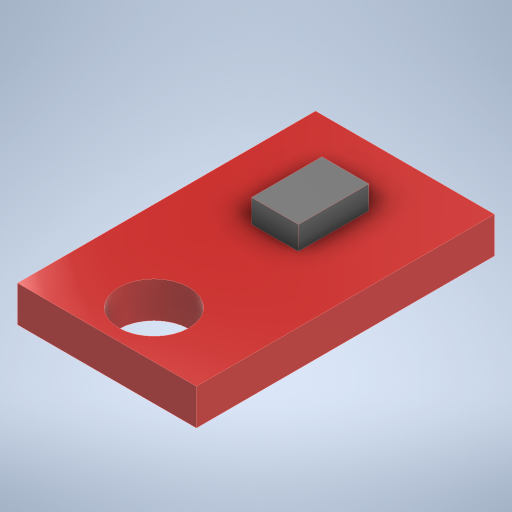
# Autodesk Inventor part: lightSensor
Saved by Autodesk Inventor 2024 (Build 280153000, 153)
## iProperties
Created: 2023-10-20
Part Number: lightSensor
Material: Generic
Document SubType Name: Modeling
Designer: kdcao
Density: 1 g/cm^3
Appearance: Orange-Red
Author: kdcao
Autodesk Inventor part; units mm, degrees
ref_plane "YZ Plane" through (0, 0, 0) normal (1, 0, 0) x (0, 1, 0)
ref_plane "XZ Plane" through (0, 0, 0) normal (0, 1, 0) x (-1, 0, 0)
ref_plane "XY Plane" through (0, 0, 0) normal (0, 0, 1) x (1, 0, 0)
sketch "Sketch1" plane through (0, 0, 0) normal (0, 1, 0) x (-1, 0, 0)
  line L0 (-3.81, 6.35) -> (3.81, 6.35)
  line L1 (3.81, 6.35) -> (3.81, -6.35)
  line L2 (3.81, -6.35) -> (-3.81, -6.35)
  line L3 (-3.81, -6.35) -> (-3.81, 6.35)
  line L4 (-3.81, 6.35) -> (3.81, -6.35) construction
  line L5 (3.81, 6.35) -> (-3.81, -6.35) construction
  point P0 (0, 0)
  dimension "d0" = 12.7
  dimension "d1" = 7.62
  constraints: 12 end point, 2 midpoint, 2 parallel, 1 horizontal, 1 perpendicular
  measures "d0" distance of L0.end L1.end
  measures "d1" distance of L0.start L0.end
extrude "Extrusion1" add sketch "Sketch1" along normal blind 2.54
sketch "Sketch2" plane through (0, 2.54, 0) normal (0, 1, 0) x (1, 0, 0)
  circle A0 centre (0, -4.35) radius 1.5
  line L0 (-3.81, -6.35) -> (3.81, -6.35) projected
  line L1 (0.9437, 3.9285) -> (-1.0563, 3.9285)
  line L2 (-1.0563, 3.9285) -> (-1.0563, 0.9285)
  line L3 (-1.0563, 0.9285) -> (0.9437, 0.9285)
  line L4 (0.9437, 0.9285) -> (0.9437, 3.9285)
  line L5 (0.9437, 3.9285) -> (-1.0563, 0.9285) construction
  line L6 (-1.0563, 3.9285) -> (0.9437, 0.9285) construction
  point P0 (0, 0)
  point P1 (0, -6.35)
  point P2 (-0.0563, 2.4285)
  dimension "d4" = 3
  dimension "d5" = 2
  dimension "d6" = 3
  dimension "d7" = 2
  constraints: 12 end point, 3 midpoint, 2 parallel, 1 centre point, 1 horizontal, 1 perpendicular
  measures "d4" diameter of A0
  measures "d5" distance of point (0, -6.35) A0.centre
  measures "d6" distance of L1.end L2.end
  measures "d7" distance of L1.start L1.end
extrude "Extrusion2" cut sketch "Sketch2" against normal through all contours A0
sketch "Sketch3" plane through (0, 2.54, 0) normal (0, 1, 0) x (1, 0, 0)
  line L0 (1.01, 0.8) -> (-0.99, 0.8)
  line L1 (-0.99, 0.8) -> (-0.99, 3.8)
  line L2 (-0.99, 3.8) -> (1.01, 3.8)
  line L3 (1.01, 3.8) -> (1.01, 0.8)
  line L4 (1.01, 0.8) -> (-0.99, 3.8) construction
  line L5 (-0.99, 0.8) -> (1.01, 3.8) construction
  line L6 (3.81, -6.35) -> (3.81, 6.35) projected
  line L7 (-3.81, -6.35) -> (3.81, -6.35) projected
  line L8 (3.81, 6.35) -> (-3.81, 6.35) projected
  line L9 (-3.81, -6.35) -> (3.81, -6.35)
  line L10 (3.81, -6.35) -> (3.81, 6.35)
  line L11 (3.81, 6.35) -> (-3.81, 6.35)
  line L12 (-3.81, 6.35) -> (-3.81, -6.35)
  point P0 (0, 0)
  point P1 (0.01, 2.3)
  dimension "d10" = 3
  dimension "d11" = 2
  dimension "d12" = 2.3
  dimension "d13" = 3.8
  constraints: 20 end point, 4 parallel, 2 horizontal, 2 midpoint, 2 perpendicular
  measures "d10" distance of L0.end L1.end
  measures "d11" distance of L1.end L2.end
  measures "d12" vertical distance of point (0, 0) point (0.01, 2.3)
  measures "d13" distance from line of L6 point (0.01, 2.3)
extrude "Extrusion3" cut sketch "Sketch3" against normal blind 1
body "Solid1"
